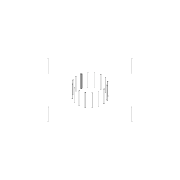
# Autodesk Inventor part: simple_ring5
Saved by Autodesk Inventor 2021 (Build 250183000, 183)
## iProperties
Created: 2022-04-11
Part Number: simple_ring5
Material: Generic
Document SubType Name: Modeling
Designer: Derm
Density: 1 g/cm^3
Appearance: Default
Author: Derm
Autodesk Inventor part; units mm, degrees
ref_plane "YZ Plane" through (0, 0, 0) normal (1, 0, 0) x (0, 1, 0)
ref_plane "XZ Plane" through (0, 0, 0) normal (0, 1, 0) x (-1, 0, 0)
ref_plane "XY Plane" through (0, 0, 0) normal (0, 0, 1) x (1, 0, 0)
sketch "Sketch1" plane through (0, 0, 0) normal (0, 1, 0) x (-1, 0, 0)
  circle A0 centre (0, 0) radius 3000 construction
  circle A1 centre (0, 0) radius 3000 construction
  circle A2 centre (0, 0) radius 3000 construction
  circle A3 centre (0, 0) radius 3000 construction
  circle A4 centre (0, 0) radius 3000 construction
  circle A5 centre (0, 0) radius 3000 construction
  circle A6 centre (0, 0) radius 3000 construction
  circle A7 centre (0, 0) radius 3000 construction
  circle A8 centre (0, 0) radius 3000 construction
  circle A9 centre (0, 0) radius 3000 construction
  circle A10 centre (0, 0) radius 3000 construction
  circle A11 centre (0, 0) radius 3000 construction
  circle A12 centre (0, 0) radius 3000 construction
  circle A13 centre (0, 0) radius 3000 construction
  circle A14 centre (0, 0) radius 3000 construction
  circle A15 centre (0, 0) radius 3000 construction
  ellipse E0 centre (2977.1789, 369.3318) end of major axis (3028.8513, 306.6592) minor radius 59.6068
  ellipse E1 centre (1480.5351, -2609.2174) end of major axis (1446.7192, -2595.3293) minor radius 17.1666
  ellipse E2 centre (798.0989, 2891.8918) end of major axis (826.7459, 2907.9915) minor radius 76.5028
  ellipse E3 centre (-2609.2174, -1480.5351) end of major axis (-2426.3157, -1555.6524) minor radius 59.9346
  ellipse E4 centre (-1480.5351, 2609.2174) end of major axis (-1517.3236, 2519.6418) minor radius 95.611
  ellipse E5 centre (2609.2174, 1480.5351) end of major axis (2564.2312, 1480.5351) minor radius 108.5183
  ellipse E6 centre (2366.3404, -1844.0263) end of major axis (2375.7265, -1845.7333) minor radius 56.5144
  line L0 (2884.6078, -635.5171) -> (3044.2654, -740.9309)
  line L1 (3044.2654, -740.9309) -> (2993.3479, -925.349)
  line L2 (2993.3479, -925.349) -> (2802.2215, -933.9118)
  line L3 (2802.2215, -933.9118) -> (2735.0164, -754.7858)
  line L4 (2735.0164, -754.7858) -> (2884.6078, -635.5171)
  ellipse E7 centre (-2977.1789, -369.3318) end of major axis (-2912.8541, -456.9927) minor radius 81.2585
  circle A16 centre (10000, 0) radius 29.4088
  circle A17 centre (0, 10000) radius 29.4088
  circle A18 centre (-10000, 0) radius 29.4088
  circle A19 centre (0, -10000) radius 29.4088
  circle A20 centre (1844.0263, 2366.3404) radius 70.7666
  circle A21 centre (-2366.3404, 1844.0263) radius 55.0542
  circle A22 centre (369.3318, -2977.1789) radius 67.2342
  circle A23 centre (-798.0989, -2891.8918) radius 52.8901
  circle A24 centre (-1844.0263, -2366.3404) radius 88.9601
  circle A25 centre (-2891.8918, 798.0989) radius 37.0023
  ellipse E8 centre (-369.3318, 2977.1789) end of major axis (-345.4922, 2866.9802) minor radius 40.3117
  point P0 (2891.8918, -798.0989)
  point P1 (2891.8918, -798.0989)
  dimension "d0" = 6000
  dimension "d3" = 360
  dimension "d7" = 10000
  dimension "d10" = 360
  constraints: 19 coincident, 16 centre point, 10 end point, 123 other
  measures "d7" distance of point (0, 0) A16.centre
extrude "Extrusion1" add sketch "Sketch1" along normal mid plane 3000
body "Solid1"
